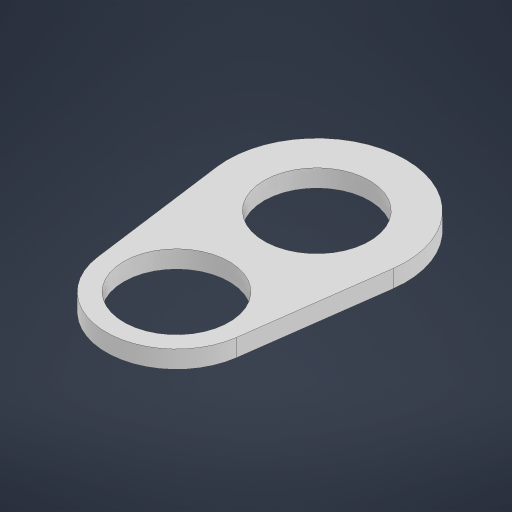
# Autodesk Inventor part: Train_006_Gearbox1
Saved by Autodesk Inventor 2024.3 (Build 283343000, 343)
## iProperties
Created: 2026-06-14
Part Number: Train_006_Gearbox1
Material: Generic
Document SubType Name: Modeling
Designer: scott
Density: 1 g/cm^3
Appearance: Default
Author: scott
Autodesk Inventor part; units mm, degrees
ref_plane "YZ Plane" through (0, 0, 0) normal (1, 0, 0) x (0, 1, 0)
ref_plane "XZ Plane" through (0, 0, 0) normal (0, 1, 0) x (-1, 0, 0)
ref_plane "XY Plane" through (0, 0, 0) normal (0, 0, 1) x (1, 0, 0)
sketch "Sketch1" plane through (0, 0, 0) normal (0, 1, 0) x (-1, 0, 0)
  circle A0 centre (0, 0) radius 15.24 construction
  circle A1 centre (0, 0) radius 16.51 construction
  circle A2 centre (0, -38.1) radius 22.86 construction
  circle A3 centre (0, -38.1) radius 24.13 construction
  circle A4 centre (0, 0) radius 14.2875
  circle A5 centre (0, -38.1) radius 14.2875
  circle A6 centre (0, 0) radius 19.05 construction
  circle A7 centre (0, -38.1) radius 24.13 construction
  line L0 (18.8799, 2.54) -> (23.9145, -34.8827)
  line L1 (-18.8799, 2.54) -> (-23.9145, -34.8827)
  arc A8 (18.8799, 2.54) -> (-18.8799, 2.54) centre (0, 0) ccw
  arc A9 (-23.9145, -34.8827) -> (23.9145, -34.8827) centre (0, -38.1) ccw
  dimension "d0" = 30.48
  dimension "d2" = 1.27
  dimension "d3" = 45.72
  dimension "d5" = 1.27
  dimension "d6" = 28.575
  dimension "d7" = 4.7625
  dimension "d8" = 1.27
  constraints: 10 centre point, 8 point on circle, 5 coincident, 5 tangent, 4 end point, 3 equal radius, 1 vertical alignment
  measures "d0" diameter of A0
  measures "d2" radial gap between concentric circles of A1 A0
  measures "d3" diameter of A2
  measures "d5" radial gap between concentric circles of A3 A2
  measures "d6" diameter of A4
  measures "d7" radial gap between concentric circles of A4 A6
  measures "d8" radial gap between concentric circles of A2 A7
extrude "Extrusion1" add sketch "Sketch1" along normal blind 4.7625
body "Solid1"
